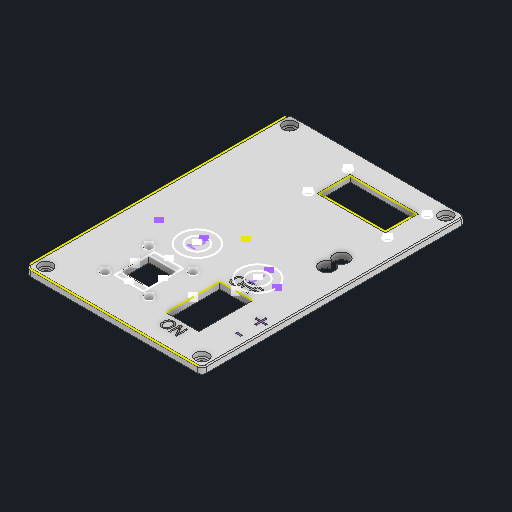
# Autodesk Inventor part: PCB_Housing_06_V4
Saved by Autodesk Inventor 2026.2 (Build 302298000, 298)
## iProperties
Created: 2026-03-17
Part Number: PCB_Housing_06_V4
Material: Generic
Document SubType Name: Modeling
Designer: vckot
Density: 1 g/cm^3
Appearance: Default
Author: vckot
Autodesk Inventor part; units mm, degrees
ref_plane "YZ Plane" through (0, 0, 0) normal (1, 0, 0) x (0, 1, 0)
ref_plane "XZ Plane" through (0, 0, 0) normal (0, 1, 0) x (-1, 0, 0)
ref_plane "XY Plane" through (0, 0, 0) normal (0, 0, 1) x (1, 0, 0)
sketch "Sketch1" plane through (0, 0, 0) normal (0, 1, 0) x (-1, 0, 0)
  line L0 (-40, 60) -> (40, 60)
  line L1 (40, 60) -> (40, -60)
  line L2 (40, -60) -> (-40, -60)
  line L3 (-40, -60) -> (-40, 60)
  line L4 (-40, 60) -> (40, -60) construction
  line L5 (40, 60) -> (-40, -60) construction
  point P0 (0, 0)
  dimension "d0" = 120
  dimension "d1" = 80
  constraints: 12 end point, 2 midpoint, 2 parallel, 1 horizontal, 1 perpendicular
  measures "d0" distance of L0.end L1.end
  measures "d1" distance of L0.start L0.end
extrude "Extrusion1" add sketch "Sketch1" along normal blind 3
sketch "Sketch2" plane through (0, 3, 0) normal (0, 1, 0) x (1, 0, 0)
  circle A0 centre (35.5, 55.5) radius 2.25
  circle A1 centre (-35.5, -55.5) radius 2.25
  arc A2 (37.5, -54.469224) -> (34.469224, -57.5) centre (35.5, -55.5) ccw
  circle A3 centre (-35.5, 55.5) radius 2.25
  circle A4 centre (35.5, -55.5) radius 2.25
  point P0 (0, 0)
  constraints: 2 centre point, 2 horizontal alignment, 2 vertical alignment
hole "Hole1" at (35.5, 3, -55.5) at (-35.5, 3, 55.5) at (35.5, 3, 55.5) at (-35.5, 3, -55.5) direction (0, -1, 0) diameter 3.75 depth 8 tip angle 118 counterbore diameter 6 counterbore depth 2
sketch "Sketch3" plane through (0, 3, 0) normal (0, 1, 0) x (1, 0, 0)
  line L0 (24.241, -45.543499) -> (24.241, -22.556499)
  line L1 (10.779, -45.543499) -> (24.241, -45.543499)
  line L2 (10.779, -22.556499) -> (10.779, -45.543499)
  line L3 (10.779, -22.556499) -> (24.241, -22.556499)
  arc A0 (26.856832, 17.449996) -> (30.143167, 17.449996) centre (28.499999, 14.999996) ccw
  arc A1 (26.856832, 10.949996) -> (30.143167, 10.949996) centre (28.499999, 8.499996) ccw
  circle A2 centre (28.499999, 8.499996) radius 2.95
  circle A3 centre (28.499999, 14.999996) radius 2.95
  line L4 (28, 35.5) -> (-2, 35.5)
  line L5 (-2, 35.5) -> (-2, 49.5)
  line L6 (-2, 49.5) -> (28, 49.5)
  line L7 (28, 49.5) -> (28, 35.5)
  circle A4 centre (-7, 34) radius 1.1
  circle A5 centre (30, 34) radius 1.1
  circle A6 centre (30, 52) radius 1.1
  circle A7 centre (-7, 52) radius 1.1
  line L8 (31.5, 32.5) -> (31.5, 53.5)
  line L9 (31.5, 53.5) -> (-8.5, 53.5)
  line L10 (-8.5, 53.5) -> (-8.5, 32.5)
  line L11 (-8.5, 32.5) -> (31.5, 32.5)
  line L12 (24.241, -22.556499) -> (10.779, -22.556499)
  line L13 (10.779, -22.556499) -> (10.779, -45.543499)
  line L14 (10.779, -45.543499) -> (24.241, -45.543499)
  line L15 (24.241, -45.543499) -> (24.241, -22.556499)
  arc A8 (12.1379, -23.305799) -> (11.7569, -23.686799) centre (12.1379, -23.686799) ccw
  line L16 (11.7569, -23.686799) -> (11.7569, -23.153399)
  line L17 (11.7569, -23.153399) -> (23.2631, -23.153399)
  line L18 (23.2631, -23.153399) -> (23.2631, -23.686799)
  arc A9 (23.2631, -23.686799) -> (22.8821, -23.305799) centre (22.8821, -23.686799) ccw
  line L19 (22.8821, -23.305799) -> (20.05, -23.305799)
  line L20 (20.05, -23.305799) -> (20.05, -23.559799)
  line L21 (20.05, -23.559799) -> (14.97, -23.559799)
  line L22 (14.97, -23.559799) -> (14.97, -23.305799)
  line L23 (14.97, -23.305799) -> (12.1379, -23.305799)
  line L24 (18.790769, -42.147052) -> (18.797824, -42.147052)
  line L25 (18.797824, -42.147052) -> (19.407999, -41.186537)
  line L26 (19.407999, -41.186537) -> (20.174294, -41.186537)
  line L27 (20.174294, -41.186537) -> (19.317111, -42.295346)
  line L28 (19.317111, -42.295346) -> (19.71607, -43.707864)
  line L29 (19.71607, -43.707864) -> (18.921553, -43.707864)
  line L30 (18.921553, -43.707864) -> (18.739263, -42.870885)
  line L31 (18.739263, -42.870885) -> (18.595587, -43.065169)
  line L32 (18.595587, -43.065169) -> (18.458966, -43.707864)
  line L33 (18.458966, -43.707864) -> (17.828648, -43.707864)
  line L34 (17.828648, -43.707735) -> (17.358303, -43.707735)
  line L35 (17.358303, -43.707735) -> (17.312378, -43.618194)
  spline S0 degree 3 poles (17.312378, -43.618194) (17.183262, -43.69882) (17.011235, -43.7391) (16.883594, -43.7391) knots 0 0 0 0 1 1 1 1
  spline S1 degree 3 poles (16.883594, -43.7391) (16.666279, -43.7391) (16.455181, -43.56555) (16.493385, -43.215144) (16.643637, -42.986824) (16.809283, -42.872511) (16.900399, -42.827654) knots 0.00500991 0.00500991 0.00500991 0.00500991 0.25104614 0.49708236 0.74311859 0.98915482 0.98915482 0.98915482 0.98915482
  spline S2 degree 3 poles (16.900399, -42.827654) (16.834462, -42.726888) (16.785779, -42.608163) (16.814322, -42.473787) knots 0 0 0 0 1 1 1 1
  spline S3 degree 3 poles (16.814322, -42.473787) (16.865314, -42.234156) (17.088333, -42.0908) (17.343615, -42.0908) knots 0 0 0 0 1 1 1 1
  spline S4 degree 3 poles (17.343615, -42.0908) (17.467218, -42.0908) (17.681137, -42.129323) (17.798163, -42.294936) (17.752062, -42.538795) (17.638072, -42.718098) (17.498782, -42.813553) (17.399546, -42.881404) knots 0.00821535 0.00821535 0.00821535 0.00821535 0.2540357 0.49985605 0.62276622 0.74567639 0.99149674 0.99149674 0.99149674 0.99149674
  line L36 (17.399546, -42.881404) -> (17.51019, -43.09865)
  spline S5 degree 3 poles (17.51019, -43.09865) (17.548931, -43.042655) (17.587672, -42.98666) (17.601014, -42.92393) knots 0 0 0 0 1 1 1 1
  line L37 (17.601014, -42.92393) -> (17.91933, -42.92393)
  line L38 (17.91933, -42.92393) -> (18.288607, -41.186537)
  line L39 (18.288607, -41.186537) -> (18.994866, -41.186537)
  line L40 (18.994866, -41.186537) -> (18.790769, -42.147052)
  line L41 (16.779109, -42.103629) -> (16.094081, -42.103629)
  line L42 (16.094081, -42.103629) -> (16.137569, -41.898762)
  spline S6 degree 3 poles (16.137569, -41.898762) (16.160852, -41.789337) (16.203698, -41.588062) (16.058867, -41.588062) knots 0 0 0 0 1 1 1 1
  spline S7 degree 3 poles (16.058867, -41.588062) (15.875231, -41.588062) (15.841172, -41.715125) (15.688773, -42.432031) knots 0 0 0 0 1 1 1 1
  spline S8 degree 3 poles (15.688773, -42.432031) (15.531947, -43.17004) (15.527073, -43.275937) (15.700062, -43.275937) knots 0 0 0 0 1 1 1 1
  spline S9 degree 3 poles (15.700062, -43.275937) (15.813078, -43.275937) (15.883056, -43.162984) (15.949827, -42.848693) knots 0 0 0 0 1 1 1 1
  line L43 (15.949827, -42.848693) -> (15.99107, -42.654473)
  line L44 (15.99107, -42.654473) -> (16.676162, -42.654473)
  line L45 (16.676162, -42.654473) -> (16.642424, -42.813415)
  spline S10 degree 3 poles (16.642424, -42.813415) (16.517028, -43.403065) (16.20838, -43.742115) (15.590444, -43.742115) knots 0.00895212 0.00895212 0.00895212 0.00895212 0.99175551 0.99175551 0.99175551 0.99175551
  spline S11 degree 3 poles (15.590444, -43.742115) (15.27401, -43.742115) (14.887863, -43.619986) (14.820678, -43.200507) (14.894815, -42.739756) (15.015532, -42.174372) (15.128196, -41.693261) (15.356087, -41.359939) (15.610614, -41.189827) (15.990864, -41.109001) (16.642583, -41.140034) (16.885652, -41.421424) (16.852223, -41.758005) (16.818145, -41.919923) knots 0.00651356 0.00651356 0.00651356 0.00651356 0.12992302 0.25333248 0.31503721 0.37674194 0.5001514 0.56185613 0.62356086 0.68526559 0.74697032 0.87037978 0.98786975 0.98786975 0.98786975 0.98786975
  line L46 (16.818171, -41.919928) -> (16.779109, -42.103629)
  line L47 (14.5255, -39.993599) -> (14.5255, -28.106399)
  line L48 (14.5255, -28.106399) -> (20.4945, -28.106399)
  line L49 (20.4945, -28.106399) -> (20.4945, -39.993599)
  line L50 (20.4945, -39.993599) -> (14.5255, -39.993599)
  arc A10 (22.8821, -44.794199) -> (23.2631, -44.413199) centre (22.8821, -44.413199) ccw
  line L51 (23.2631, -44.413199) -> (23.2631, -44.946599)
  line L52 (23.2631, -44.946599) -> (11.7569, -44.946599)
  line L53 (11.7569, -44.946599) -> (11.7569, -44.413199)
  arc A11 (11.7569, -44.413199) -> (12.1379, -44.794199) centre (12.1379, -44.413199) ccw
  line L54 (12.1379, -44.794199) -> (22.8821, -44.794199)
  point P0 (0, 0)
  point P1 (26.856832, 10.949996)
extrude "Extrusion2" cut sketch "Sketch3" against normal through all contours L1 L2 L3 L0 | A3 A0 | A2 A1 | L4 L5 L6 L7 | A8 L16 L17 L18 A9 L19 L20 L21 L22 L23 | L24 L25 L26 L27 L28 L29 L30 L31 L32 L33 L34 L35 S0 S1 S2 S3 S4 L36 S5 L37 L38 L39 L40 | L41 L42 S6 S7 S8 S9 L43 L44 L45 S10 S11 L46 | L47 L48 L49 L50 | A10 L51 L52 L53 A11 L54
sketch "Sketch5" plane through (0, 3, 0) normal (0, 1, 0) x (1, 0, 0)
  circle A0 centre (-5, 33.5) radius 1.75
  circle A1 centre (-5, 51.5) radius 1.75
  circle A2 centre (31, 51.5) radius 1.75
  circle A3 centre (31, 33.5) radius 1.75
  line L0 (28, 35.5) -> (-2, 35.5) projected
  line L1 (-2, 35.5) -> (-2, 49.5) projected
  line L2 (-2, 49.5) -> (28, 49.5) projected
  line L3 (28, 49.5) -> (28, 35.5) projected
  point P0 (0, 0)
  dimension "d27" = 3.5
  dimension "d28" = 2
  dimension "d29" = 3
  dimension "d30" = 2
  dimension "d31" = 3
  dimension "d32" = 3
  dimension "d33" = 3
  dimension "d34" = 2
  dimension "d35" = 2
  constraints: 4 centre point, 3 equal radius
  measures "d27" diameter of A0
  measures "d28" distance from line of A0.centre L0
  measures "d29" distance from line of L1 A0.centre
  measures "d30" distance from line of L2 A1.centre
  measures "d31" distance from line of L1 A1.centre
  measures "d32" distance from line of L3 A2.centre
  measures "d33" distance from line of L3 A3.centre
  measures "d34" distance from line of L0 A3.centre
  measures "d35" distance from line of L2 A2.centre
thicken "Thicken1" operation add thickness 0.5 both sides no extend neighbours yes toward (0, 0, -1) faces at (18, 2, -49.5) (-2, 2, -44.833333) (28, 2, -40.166667) (8, 2, -35.5)
thicken "Thicken2" operation add thickness 0.5 both sides no extend neighbours yes toward (0.6830158, 0, -0.7304036) faces at (30.514896, 2, -17.154687)
thicken "Thicken3" operation add thickness 0.5 both sides no extend neighbours yes toward (0.6830158, 0, -0.7304036) faces at (30.514896, 2, -10.654687)
thicken "Thicken4" operation add thickness 0.75 both sides no extend neighbours yes toward (1, 0, 0) faces at (24.241, 2, 37.881166) (15.266333, 1, 22.556499) (10.779, 2, 30.218832) (15.266333, 2, 45.543499)
sketch "Sketch4" plane through (0, 3, 0) normal (0, 1, 0) x (1, 0, 0)
  line L0 (7.168033, -20.561799) -> (27.698693, -20.561798) construction
  line L1 (27.698693, -20.561798) -> (27.698693, -47.5382) construction
  line L2 (27.698693, -47.5382) -> (7.168033, -47.5382) construction
  line L3 (7.168033, -47.5382) -> (7.168033, -20.561799) construction
  line L4 (10.029, -21.806499) -> (24.991, -21.806499)
  line L5 (10.029, -46.293499) -> (10.029, -21.806499)
  spline S0 degree 2 poles (15.458079, -15.656575) (15.741709, -15.988828) (16.057755, -16.961276) (16.057755, -17.585263) knots 0 0 0 1 2 2 2
  spline S1 degree 2 poles (16.057755, -17.585263) (16.057755, -18.193042) (15.749813, -19.177645) (15.458079, -19.509898) knots 0 0 0 1 2 2 2
  spline S2 degree 2 poles (15.458079, -19.509898) (15.150137, -19.858358) (14.335713, -20.190611) (13.845437, -20.190611) knots 0 0 0 1 2 2 2
  spline S3 degree 2 poles (13.845437, -20.190611) (13.338954, -20.190611) (12.528582, -19.846203) (12.232795, -19.509898) knots 0 0 0 1 2 2 2
  spline S4 degree 2 poles (12.232795, -19.509898) (11.945113, -19.177645) (11.637171, -18.201146) (11.637171, -17.585263) knots 0 0 0 1 2 2 2
  spline S5 degree 2 poles (11.637171, -17.585263) (11.637171, -16.957224) (11.949165, -16.000984) (12.236847, -15.656576) knots 0 0 0 1 2 2 2
  spline S6 degree 2 poles (12.236847, -15.656576) (12.528581, -15.324323) (13.343006, -14.979914) (13.845437, -14.979914) knots 0 0 0 1 2 2 2
  spline S7 degree 2 poles (13.845437, -14.979914) (14.355972, -14.979914) (15.174449, -15.336478) (15.458079, -15.656575) knots 0 0 0 1 2 2 2
  spline S8 degree 2 poles (15.364886, -17.585263) (15.364886, -17.090935) (15.150137, -16.325133) (14.955648, -16.073917) knots 0 0 0 1 2 2 2
  spline S9 degree 2 poles (14.955648, -16.073917) (14.757107, -15.814598) (14.197949, -15.555279) (13.849489, -15.555279) knots 0 0 0 1 2 2 2
  spline S10 degree 2 poles (13.849489, -15.555279) (13.488873, -15.555279) (12.945923, -15.806495) (12.739278, -16.073918) knots 0 0 0 1 2 2 2
  spline S11 degree 2 poles (12.739278, -16.073918) (12.540737, -16.329185) (12.33004, -17.099039) (12.33004, -17.585263) knots 0 0 0 1 2 2 2
  spline S12 degree 2 poles (12.33004, -17.585263) (12.33004, -18.569866) (13.15662, -19.615247) (13.849489, -19.615247) knots 0 0 0 1 2 2 2
  spline S13 degree 2 poles (13.849489, -19.615247) (14.542358, -19.615247) (15.364886, -18.569866) (15.364886, -17.585263) knots 0 0 0 1 2 2 2
  line L6 (19.777366, -15.676835) -> (17.451596, -15.676835)
  line L7 (17.451596, -15.676835) -> (17.451596, -17.086883)
  line L8 (17.451596, -17.086883) -> (19.680121, -17.086883)
  line L9 (19.680121, -17.086883) -> (19.680121, -17.678455)
  line L10 (19.680121, -17.678455) -> (17.451596, -17.678456)
  line L11 (17.451596, -17.678456) -> (17.451596, -20.085263)
  line L12 (17.451596, -20.085263) -> (16.78709, -20.085263)
  line L13 (16.78709, -20.085263) -> (16.78709, -15.085263)
  line L14 (16.78709, -15.085263) -> (19.777366, -15.085263)
  line L15 (19.777366, -15.085263) -> (19.777366, -15.676835)
  line L16 (23.363265, -15.676835) -> (21.037496, -15.676835)
  line L17 (21.037496, -15.676835) -> (21.037496, -17.086883)
  line L18 (21.037496, -17.086883) -> (23.266021, -17.086883)
  line L19 (23.266021, -17.086883) -> (23.266021, -17.678455)
  line L20 (23.266021, -17.678455) -> (21.037496, -17.678455)
  line L21 (21.037496, -17.678455) -> (21.037496, -20.085263)
  line L22 (21.037496, -20.085263) -> (20.37299, -20.085263)
  line L23 (20.37299, -20.085263) -> (20.37299, -15.085263)
  line L24 (20.37299, -15.085263) -> (23.363265, -15.085263)
  line L25 (23.363265, -15.085263) -> (23.363265, -15.676835)
  spline S14 degree 2 poles (16.748599, -48.586048) (17.032229, -48.918301) (17.348275, -49.890749) (17.348275, -50.514736) knots 0 0 0 1 2 2 2
  spline S15 degree 2 poles (17.348275, -50.514736) (17.348275, -51.122515) (17.040333, -52.107118) (16.748599, -52.439371) knots 0 0 0 1 2 2 2
  spline S16 degree 2 poles (16.748599, -52.439371) (16.440657, -52.787831) (15.626232, -53.120084) (15.135957, -53.120084) knots 0 0 0 1 2 2 2
  spline S17 degree 2 poles (15.135957, -53.120084) (14.629474, -53.120084) (13.819101, -52.775676) (13.523315, -52.439371) knots 0 0 0 1 2 2 2
  spline S18 degree 2 poles (13.523315, -52.439371) (13.235633, -52.107118) (12.927691, -51.130619) (12.927691, -50.514736) knots 0 0 0 1 2 2 2
  spline S19 degree 2 poles (12.927691, -50.514736) (12.927691, -49.886697) (13.239685, -48.930457) (13.527367, -48.586048) knots 0 0 0 1 2 2 2
  spline S20 degree 2 poles (13.527367, -48.586048) (13.819101, -48.253796) (14.633526, -47.909387) (15.135957, -47.909387) knots 0 0 0 1 2 2 2
  spline S21 degree 2 poles (15.135957, -47.909387) (15.646492, -47.909387) (16.464968, -48.265951) (16.748599, -48.586048) knots 0 0 0 1 2 2 2
  spline S22 degree 2 poles (16.655406, -50.514736) (16.655406, -50.020408) (16.440657, -49.254606) (16.246168, -49.00339) knots 0 0 0 1 2 2 2
  spline S23 degree 2 poles (16.246168, -49.00339) (16.047626, -48.744071) (15.488469, -48.484752) (15.140009, -48.484752) knots 0 0 0 1 2 2 2
  spline S24 degree 2 poles (15.140009, -48.484752) (14.779393, -48.484752) (14.236443, -48.735967) (14.029798, -49.00339) knots 0 0 0 1 2 2 2
  spline S25 degree 2 poles (14.029798, -49.00339) (13.831257, -49.258658) (13.62056, -50.028512) (13.62056, -50.514736) knots 0 0 0 1 2 2 2
  spline S26 degree 2 poles (13.62056, -50.514736) (13.62056, -51.499339) (14.44714, -52.544719) (15.140009, -52.544719) knots 0 0 0 1 2 2 2
  spline S27 degree 2 poles (15.140009, -52.544719) (15.832877, -52.544719) (16.655406, -51.499339) (16.655406, -50.514736) knots 0 0 0 1 2 2 2
  line L26 (21.655406, -53.014735) -> (20.909863, -53.014735)
  line L27 (20.909863, -53.014735) -> (18.697545, -48.703552)
  line L28 (18.697545, -48.703552) -> (18.697545, -53.014736)
  line L29 (18.697545, -53.014736) -> (18.07761, -53.014736)
  line L30 (18.07761, -53.014736) -> (18.07761, -48.014736)
  line L31 (18.07761, -48.014736) -> (19.021694, -48.014736)
  line L32 (19.021694, -48.014736) -> (21.035471, -51.973406)
  line L33 (21.035471, -51.973406) -> (21.035471, -48.014735)
  line L34 (21.035471, -48.014735) -> (21.655406, -48.014735)
  line L35 (21.655406, -48.014735) -> (21.655406, -53.014735)
  point P0 (0, 0)
  point P1 (27.698693, -34.049999)
  point P2 (10.029, -34.049999)
  dimension "d0" = 120
  dimension "d1" = 80
  constraints: 2 midpoint, 1 horizontal alignment, 2 other
extrude "Extrusion3" cut sketch "Sketch4" against normal blind 2
fillet "Fillet1" radius 2 4 edges at (-40, 1.5, -60) (-40, 1.5, 60) (40, 1.5, -60) (40, 1.5, 60)
fillet "Fillet2" radius 0.5 8 edges at (39.4142, 3, -59.4142) (0, 3, -60) (-39.4142, 3, -59.4142) (-40, 3, 0) (-39.4142, 3, 59.4142) (0, 3, 60) (39.4142, 3, 59.4142) (40, 3, 0)
sketch "Sketch6" plane through (0, 3, 0) normal (0, 1, 0) x (1, 0, 0)
  line L0 (8.988356, -6.885061) -> (26.031643, -6.885061) construction
  line L1 (26.031643, -6.885061) -> (26.031643, -17.114939) construction
  line L2 (26.031643, -17.114939) -> (8.988356, -17.114939) construction
  line L3 (8.988356, -17.114939) -> (8.988356, -6.885061) construction
  circle A0 centre (17.51, -12) radius 4.5
  circle A1 centre (17.51, -12) radius 8
  line L4 (10.029, -21.806499) -> (24.991, -21.806499)
  line L5 (-16.5, -25.049999) -> (-3.5, -25.049999)
  line L6 (-3.5, -25.049999) -> (-3.5, -43.049999)
  line L7 (-3.5, -43.049999) -> (-16.5, -43.049999)
  line L8 (-16.5, -43.049999) -> (-16.5, -25.049999)
  line L9 (-40, 58) -> (-40, -58)
  line L10 (-38, -60) -> (38, -60)
  line L11 (-16.5, -27.549999) -> (-3.5, -27.549999)
  line L12 (-3.5, -27.549999) -> (-3.5, -40.549999)
  line L13 (-3.5, -40.549999) -> (-16.5, -40.549999)
  line L14 (-16.5, -40.549999) -> (-16.5, -27.549999)
  circle A2 centre (-10, -12) radius 4.5
  circle A3 centre (-10, -12) radius 8
  line L15 (-27.288736, -8.885737) -> (7.288736, -8.885737) construction
  line L16 (7.288736, -8.885737) -> (7.288736, -15.114263) construction
  line L17 (7.288736, -15.114263) -> (-27.288736, -15.114263) construction
  line L18 (-27.288736, -15.114263) -> (-27.288736, -8.885737) construction
  circle A4 centre (0, -24.049999) radius 1.875
  circle A5 centre (-20, -24.049999) radius 1.875
  circle A6 centre (-20, -44.049999) radius 1.875
  circle A7 centre (0, -44.049999) radius 1.875
  line L19 (10.029, -46.293499) -> (10.029, -21.806499)
  line L20 (31.770346, -23.604815) -> (38.410651, -23.604815) construction
  line L21 (38.410651, -23.604815) -> (38.410651, -40.724353) construction
  line L22 (38.410651, -40.724353) -> (31.770346, -40.724353) construction
  line L23 (31.770346, -40.724353) -> (31.770346, -23.604815) construction
  line L24 (37.500345, -28.482466) -> (35.434056, -28.482466)
  line L25 (35.434056, -28.482466) -> (35.434056, -30.548755)
  line L26 (35.434056, -30.548755) -> (34.751884, -30.548755)
  line L27 (34.751884, -30.548755) -> (34.751884, -28.482466)
  line L28 (34.751884, -28.482466) -> (32.685596, -28.482466)
  line L29 (32.685596, -28.482466) -> (32.685596, -27.825011)
  line L30 (32.685596, -27.825011) -> (34.751884, -27.825011)
  line L31 (34.751884, -27.825011) -> (34.751884, -25.758722)
  line L32 (34.751884, -25.758722) -> (35.434056, -25.758722)
  line L33 (35.434056, -25.758722) -> (35.434056, -27.825011)
  line L34 (35.434056, -27.825011) -> (37.500345, -27.825011)
  line L35 (37.500345, -27.825011) -> (37.500345, -28.482466)
  line L36 (36.247225, -38.570445) -> (33.938716, -38.570445)
  line L37 (33.938716, -38.570445) -> (33.938716, -37.828954)
  line L38 (33.938716, -37.828954) -> (36.247225, -37.828954)
  line L39 (36.247225, -37.828954) -> (36.247225, -38.570445)
  point P0 (0, 0)
  point P1 (17.51, -21.806499)
  point P2 (-10, -43.049999)
  point P3 (-3.5, -34.049999)
  point P4 (-16.5, -34.049999)
  point P5 (-16.5, -34.049999)
  point P6 (-10, -25.049999)
  point P7 (-10, -8.885737)
  point P8 (-27.288736, -12)
  point P9 (26.031643, -12)
  point P10 (17.51, -6.885061)
  point P11 (-16.5, -40.549999)
  point P12 (-3.5, -27.549999)
  point P13 (-3.5, -34.049999)
  point P14 (10.029, -34.049999)
  dimension "d0" = 120
  dimension "d1" = 80
  dimension "d38" = 16
  dimension "d39" = 9
  dimension "d40" = 18
  dimension "d41" = 13
  dimension "d42" = 30
  dimension "d44" = 13
  dimension "d45" = 48
  dimension "d46" = 16
  dimension "d47" = 9
  dimension "d48" = 3.75
  dimension "d50" = 3.5
  dimension "d51" = 3.5
  dimension "d52" = 3.5
  dimension "d53" = 3.5
  constraints: 16 end point, 12 midpoint, 8 centre point, 6 horizontal alignment, 6 vertical alignment, 4 parallel, 3 coincident, 3 equal radius, 2 horizontal, 2 perpendicular, 2 point on line, 6 other
  measures "d38" diameter of A1
  measures "d39" diameter of A0
  measures "d40" distance between parallel lines of L7 L5
  measures "d41" distance between parallel lines of L8 L6
  measures "d42" distance from line of L9 point (-10, -43.05)
  measures "d44" distance between parallel lines of L13 L11
  measures "d45" distance from line of L10 A1.centre
  measures "d46" diameter of A3
  measures "d47" diameter of A2
  measures "d48" diameter of A4
  measures "d50" distance from line of A4.centre L11
  measures "d51" distance from line of A4.centre L12
  measures "d52" distance from line of L13 A7.centre
  measures "d53" distance from line of A6.centre L8
extrude "Extrusion5" cut sketch "Sketch6" against normal blind 2.5 contours L11 L6 L13 L8 | L24 L25 L26 L27 L28 L29 L30 L31 L32 L33 L34 L35 | L36 L37 L38 L39
extrude "Extrusion7" cut sketch "Sketch6" against normal blind 10 contours L11 L6 L13 L8 | A4 | A5 | A6 | A7
body "Solid1"
